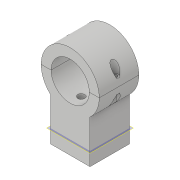
# Autodesk Inventor part: Lensagon1.2x-ThorlabsRailCarriage(XT66P2M)
Saved by Autodesk Inventor 2021 (Build 250183000, 183)
## iProperties
Created: 2022-02-11
Part Number: Lensagon1.2x-ThorlabsRailCarriage(XT66P2M)
Material: Generic
Document SubType Name: Modeling
Designer: Nikita
Density: 1 g/cm^3
Appearance: Default
Author: Nikita
Autodesk Inventor part; units mm, degrees
sketch "Sketch1" plane through (0, 0, 0) normal (0, 0, 1) x (1, 0, 0)
  circle A0 centre (0, 0) radius 27.95
  circle A1 centre (0, 0) radius 42.5
  line L0 (0, 9.3391) -> (0, -10.826)
  line L1 (10.223, 0) -> (-10.1436, 0)
  line L2 (29, -94) -> (-29, -94)
  line L3 (-29, -94) -> (-29, -31.0685)
  line L4 (-29, -31.0685) -> (29, -31.0685)
  line L5 (29, -31.0685) -> (29, -94)
  point P0 (-29, -94)
  dimension "d1" = 85
  dimension "d0" = 55.9
  dimension "d41" = 94
  constraints: 12 end point, 3 coincident, 2 horizontal, 2 parallel, 1 centre point, 1 perpendicular, 1 symmetric about line, 1 vertical, 3 other
  measures "d0" diameter of A0
  measures "d41" distance from line of L2 point (0, 0)
extrude "Extrusion1" add sketch "Sketch1" along normal blind 58
ref_plane "BoltPlane" through (0, 50, 0) normal (0, 1, 0) x (-1, 0, 0)
sketch "BoltHoles" plane through (0, 50, 0) normal (0, 1, 0) x (-1, 0, 0)
  line L0 (27.95, 0) -> (27.95, 58) projected
  line L1 (42.5, 0) -> (42.5, 58) projected
  line L2 (27.95, 0) -> (27.95, 58) projected
  line L3 (27.95, 0) -> (27.95, 58) projected
  line L4 (-42.5, 0) -> (-42.5, 58) projected
  line L5 (-27.95, 0) -> (-27.95, 58) projected
  line L6 (27.95, 0) -> (27.95, 58) projected
  line L7 (27.95, 0) -> (27.95, 58) projected
  line L8 (-27.95, 0) -> (-27.95, 58) projected
  line L9 (0, 84.6518) -> (0, 68.3892)
  circle A0 centre (36.5, 29) radius 3.2
  circle A1 centre (36.5, 29) radius 5.2
  circle A2 centre (-36.5, 29) radius 3.2
  circle A3 centre (-36.5, 29) radius 5.2
  point P0 (0, 0)
  dimension "d7" = 6
  dimension "d8" = 6.4
  dimension "d9" = 10.4
  constraints: 4 centre point, 4 coincident, 3 symmetric about line, 2 end point, 1 vertical, 4 other
  measures "d7" distance from line of L1 point (36.5, 29)
  measures "d8" diameter of A0
  measures "d9" diameter of A1
extrude "Extrusion2" cut sketch "BoltHoles" against normal through all contours A0 | A2
extrude "Extrusion3" cut sketch "BoltHoles" against normal blind 40
ref_plane "NutPlane" through (0, -80, 0) normal (0, 1, 0) x (-1, 0, 0)
sketch "NutHoles" plane through (0, -80, 0) normal (0, 1, 0) x (-1, 0, 0)
  circle A0 centre (-36.5, 29) radius 3.2 projected
  line L0 (-42.5044, 29) -> (-39.5022, 34.2)
  line L1 (-39.5022, 34.2) -> (-33.4978, 34.2)
  line L2 (-33.4978, 34.2) -> (-30.4956, 29)
  line L3 (-30.4956, 29) -> (-33.4978, 23.8)
  line L4 (-33.4978, 23.8) -> (-39.5022, 23.8)
  line L5 (-39.5022, 23.8) -> (-42.5044, 29)
  line L6 (0, 84.6518) -> (0, 68.3892) projected
  circle A1 centre (36.5, 29) radius 3.2
  line L7 (42.5044, 29) -> (39.5022, 34.2)
  line L8 (39.5022, 34.2) -> (33.4978, 34.2)
  line L9 (33.4978, 34.2) -> (30.4956, 29)
  line L10 (30.4956, 29) -> (33.4978, 23.8)
  line L11 (33.4978, 23.8) -> (39.5022, 23.8)
  line L12 (39.5022, 23.8) -> (42.5044, 29)
  line L13 (-6.5676, 29) -> (7.2641, 29)
  point P0 (0, 0)
  point P1 (0, 41.5)
  point P2 (0, 16.5)
  dimension "d15" = 10.4
  dimension "d28" = 12.5
  constraints: 26 end point, 10 symmetric about line, 2 coincident, 2 horizontal, 1 centre point, 14 other
  measures "d15" distance between parallel lines of L1 L4
  measures "d28" distance from line of point (0, 41.5) L13
extrude "Extrusion4" cut sketch "NutHoles" along normal blind 70
ref_plane "SplitPlane" through (0, 0, 0) normal (0, 1, 0) x (-1, 0, 0)
split body "Split2" result two bodies by plane through (0, 0, 0) normal (0, 1, 0) first body at (41.8684, 3.3218, 29.6612)
hole "Hole2" at (0, -80, 41.5) at (0, -80, 16.5) direction (0, -1, 0) diameter 6.2 end through all both bodies 3
sketch "Sketch4" plane through (0, 0, 0) normal (0, 1, 0) x (-1, 0, 0)
  circle A0 centre (0, 41.5) radius 5.1
  circle A1 centre (0, 16.5) radius 5.1
  point P0 (0, 0)
  dimension "d36" = 10.2
  dimension "d37" = 10.2
  constraints: 2 centre point, 2 coincident
  measures "d36" diameter of A0
  measures "d37" diameter of A1
ref_plane "BoltHeadLevel" through (0, -62, 0) normal (0, 1, 0) x (-1, 0, 0)
ref_plane "BoltHeadsPlane(35mm-M6-bolts)" through (-29, -74, 0) normal (0, -1, 0) x (1, 0, 0)
extrude "Extrusion5" cut sketch "Sketch4" against normal up to surface (74 mm away) bodies 3
